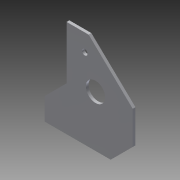
# Autodesk Inventor part: OutlineSketch1
Saved by Autodesk Inventor 2013 (Build 170138000, 138)
## iProperties
Created: 2013-06-03
Part Number: OutlineSketch1
Material: Aluminum 6061
Document SubType Name: Modeling
Designer: mvarma
Density: 1 g/cm^3
Author: mvarma
Autodesk Inventor part; units mm, degrees
ref_plane "YZ Plane" through (0, 0, 0) normal (1, 0, 0) x (0, 1, 0)
ref_plane "XZ Plane" through (0, 0, 0) normal (0, 1, 0) x (-1, 0, 0)
ref_plane "XY Plane" through (0, 0, 0) normal (0, 0, 1) x (1, 0, 0)
sketch "Sketch1" plane through (0, 0, 0) normal (0, 0, 1) x (1, 0, 0)
  line L0 (0, 0) -> (304.8, 0) construction
  line L1 (304.8, 0) -> (304.8, 50.8) construction
  line L2 (304.8, 50.8) -> (0, 50.8) construction
  line L3 (0, 50.8) -> (0, 0) construction
  circle A0 centre (152.4, 25.4) radius 14.2875 construction
  circle A1 centre (152.4, 25.4) radius 30.48 construction
  circle A2 centre (152.4, 25.4) radius 22.225 construction
  line L4 (152.4, 25.4) -> (138.5082, 62.9697) construction
  circle A3 centre (138.5082, 62.9697) radius 9.525 construction
  circle A4 centre (138.5082, 62.9697) radius 17.78 construction
  circle A5 centre (89.9711, 85.09) radius 31.75 construction
  circle A6 centre (160.9785, 111.3458) radius 31.75 construction
  circle A7 centre (221.9701, 85.09) radius 31.75 construction
  line L5 (0, 50.8) -> (0, 53.34) construction
  line L6 (0, 53.34) -> (304.8, 53.34) construction
  line L7 (304.8, 53.34) -> (304.8, 50.8) construction
  circle A8 centre (138.5082, 62.9697) radius 21.59 construction
  circle A9 centre (152.4, 25.4) radius 46.99 construction
  circle A10 centre (152.4, 25.4) radius 50.8 construction
  arc A11 (84.9408, 79.3264) -> (90.9184, 92.6811) centre (89.9711, 85.09) ccw construction
  circle A12 centre (160.9785, 111.3458) radius 7.65 construction
  arc A13 (221.6946, 92.735) -> (225.5172, 78.312) centre (221.9701, 85.09) ccw construction
  circle A14 centre (160.9785, 111.3458) radius 9.1 construction
  circle A15 centre (138.5082, 62.9697) radius 22.9 construction
  line L8 (84.9408, 79.3264) -> (123.4503, 45.7166) construction
  line L9 (168.5483, 110.2412) -> (161.1682, 59.6633) construction
  line L10 (90.9184, 92.6811) -> (89.9711, 85.09) construction
  line L11 (89.9711, 85.09) -> (84.9408, 79.3264) construction
  circle A16 centre (126.192, 96.2783) radius 3.175
  circle A17 centre (126.192, 96.2783) radius 7.9375 construction
  line L12 (90.9184, 92.6811) -> (125.2091, 88.4019) construction
  line L13 (132.0626, 90.936) -> (155.3205, 116.4945) construction
  line L14 (155.3205, 116.4945) -> (160.9785, 111.3458) construction
  line L15 (168.5483, 110.2412) -> (160.9785, 111.3458) construction
  line L16 (138.5082, 62.9697) -> (126.192, 96.2783) construction
  line L17 (89.9711, 85.09) -> (160.9785, 111.3458) construction
  line L18 (152.4, 25.4) -> (89.9711, 85.09) construction
  line L19 (152.4, 25.4) -> (160.9785, 111.3458) construction
  circle A18 centre (126.192, 96.2783) radius 9.2075 construction
  circle A19 centre (126.192, 96.2783) radius 6.1595 construction
  arc A20 (90.9184, 92.6811) -> (84.9408, 79.3264) centre (89.9711, 85.09) ccw construction
  circle A21 centre (160.9785, 111.3458) radius 25.4 construction
  circle A22 centre (221.9701, 85.09) radius 25.4 construction
  line L20 (102.9424, 114.0695) -> (76.9998, 56.1105) construction
  circle A23 centre (89.9711, 85.09) radius 25.4 construction
  line L21 (213.8361, 115.7804) -> (230.1041, 54.3996) construction
  line L22 (54.4111, 146.9058) -> (257.6111, 146.9058)
  line L23 (257.6111, 146.9058) -> (257.6111, -11.8442)
  line L24 (257.6111, -11.8442) -> (54.4111, -11.8442)
  line L25 (54.4111, -11.8442) -> (54.4111, 146.9058)
  circle A24 centre (138.5082, 62.9697) radius 11.1125
  arc A25 (225.3129, 75.4455) -> (221.0936, 95.3227) centre (223.2033, 85.3841) ccw construction
  line L26 (220.7531, 84.7347) -> (228.4773, 60.5377) construction
  line L27 (223.2033, 85.3841) -> (228.4773, 60.5377) construction
  line L28 (220.7531, 84.7347) -> (213.029, 108.9318) construction
  line L29 (223.2033, 85.3841) -> (217.9292, 110.2305) construction
  arc A26 (212.3049, 111.2003) -> (213.7531, 106.6633) centre (213.029, 108.9318) ccw construction
  arc A27 (218.4237, 107.9012) -> (217.4348, 112.5599) centre (217.9292, 110.2305) ccw construction
  arc A28 (218.4237, 107.9012) -> (213.7531, 106.6633) centre (228.4773, 60.5377) ccw construction
  arc A29 (217.4348, 112.5599) -> (212.3049, 111.2003) centre (228.4773, 60.5377) ccw construction
  line L30 (213.029, 108.9318) -> (212.3049, 111.2003) construction
  line L31 (217.9292, 110.2305) -> (217.4348, 112.5599) construction
  arc A30 (221.0936, 95.3227) -> (217.6635, 94.4136) centre (228.4773, 60.5377) ccw construction
  arc A31 (225.3129, 75.4455) -> (223.8428, 75.0559) centre (228.4773, 60.5377) ccw construction
  line L32 (102.6358, 107.1803) -> (91.1149, 84.5434) construction
  line L33 (79.5941, 61.9064) -> (88.8014, 85.5789) construction
  arc A32 (98.8719, 111.4706) -> (97.1455, 107.0321) centre (98.0087, 109.2513) ccw construction
  arc A33 (101.5557, 105.0581) -> (103.7158, 109.3025) centre (102.6358, 107.1803) ccw construction
  arc A34 (101.5557, 105.0581) -> (97.1455, 107.0321) centre (79.5941, 61.9064) ccw construction
  line L34 (98.0087, 109.2513) -> (98.8719, 111.4706) construction
  line L35 (102.6358, 107.1803) -> (103.7158, 109.3025) construction
  arc A35 (103.7158, 109.3025) -> (98.8719, 111.4706) centre (79.5941, 61.9064) ccw construction
  arc A36 (217.6635, 94.4136) -> (223.8428, 75.0559) centre (220.7531, 84.7347) ccw construction
  arc A37 (86.5066, 75.4886) -> (95.7233, 93.5981) centre (91.1149, 84.5434) ccw construction
  line L36 (88.8014, 85.5789) -> (98.0087, 109.2513) construction
  line L37 (91.1149, 84.5434) -> (79.5941, 61.9064) construction
  arc A38 (86.5066, 75.4886) -> (85.1185, 76.1099) centre (79.5941, 61.9064) ccw construction
  arc A39 (95.7233, 93.5981) -> (92.4843, 95.0479) centre (79.5941, 61.9064) ccw construction
  arc A40 (92.4843, 95.0479) -> (85.1185, 76.1099) centre (88.8014, 85.5789) ccw construction
  line L38 (160.9785, 111.3458) -> (138.0151, 122.2014) construction
  line L39 (160.9785, 111.3458) -> (183.9418, 100.4902) construction
  circle A41 centre (138.5082, 62.9697) radius 26.75 construction
  line L40 (221.6946, 92.735) -> (137.5448, 89.7024) construction
  line L41 (225.5172, 78.312) -> (150.9113, 39.269) construction
  line L42 (221.9701, 85.09) -> (221.6946, 92.735) construction
  line L43 (221.9701, 85.09) -> (225.5172, 78.312) construction
  line L44 (138.5082, 62.9697) -> (137.5448, 89.7024) construction
  line L45 (138.5082, 62.9697) -> (150.9113, 39.269) construction
  arc A42 (225.5172, 78.312) -> (221.6946, 92.735) centre (221.9701, 85.09) ccw construction
  arc A43 (225.5172, 78.312) -> (224.7763, 77.9733) centre (221.9701, 85.09) ccw construction
  line L46 (138.5082, 62.9697) -> (221.9701, 85.09) construction
  line L47 (79.8111, 29.4308) -> (105.2111, 54.8308)
  line L48 (105.2111, 54.8308) -> (105.2111, 116.102)
  line L49 (105.2111, 116.102) -> (130.6111, 116.102)
  line L50 (130.6111, 116.102) -> (181.4111, 67.5308)
  line L51 (181.4111, 67.5308) -> (181.4111, 29.4308)
  line L52 (156.0111, 4.0308) -> (79.8111, 4.0308)
  line L53 (79.8111, 4.0308) -> (79.8111, 29.4308)
  line L54 (156.0111, 4.0308) -> (181.4111, 29.4308)
  point P0 (215.4629, 109.6423)
  point P1 (100.3481, 108.2736)
  dimension "d1" = 50.8
  dimension "d2" = 28.575
  dimension "d3" = 25.4
  dimension "d4" = 152.4
  dimension "d7" = 60.96
  dimension "d8" = 44.45
  dimension "d9" = 19.05
  dimension "d10" = 35.56
  dimension "d11" = 40.0558
  dimension "d12" = 63.5
  dimension "d13" = 63.5
  dimension "d14" = 63.5
  dimension "d15" = 2.54
  dimension "d16" = 304.8
  dimension "d17" = 43.18
  dimension "d18" = 93.98
  dimension "d19" = 101.6
  dimension "d21" = 15.3
  dimension "d22" = 15.3
  dimension "d24" = 18.2
  dimension "d29" = 45.8
  dimension "d30" = 146
  dimension "d31" = 6.35
  dimension "d32" = 15.875
  dimension "d33" = 146
  dimension "d35" = 18.415
  dimension "d37" = 12.319
  dimension "d40" = 50.8
  dimension "d41" = 50.8
  dimension "d42" = 17
  dimension "d43" = 17
  dimension "d44" = 50.8
  dimension "d53" = 203.2
  dimension "d54" = 158.75
  dimension "d55" = 35.56
  dimension "d56" = 35.56
  dimension "d57" = 22.225
  dimension "d67" = 25.4
  dimension "d68" = 25.4
  dimension "d69" = 2.86
  dimension "d70" = 25.4
  dimension "d71" = 25.4
  dimension "d72" = 4.7625
  dimension "d75" = 2.86
  dimension "d80" = 4.7625
  dimension "d82" = 4.7625
  dimension "d83" = 50.8
  dimension "d84" = 50.8
  dimension "d85" = 10.16
  dimension "d97" = 48.4188
  dimension "d99" = 20.32
  dimension "d101" = 25.4
  dimension "d102" = 25.4
  dimension "d103" = 10.16
  dimension "d105" = 17
  dimension "d106" = 17
  dimension "d107" = 53.5
  dimension "d108" = 154.44
  dimension "d109" = 7.65
  dimension "d111" = 86.3435
  dimension "d112" = 12.78
  dimension "d113" = 12.78
  dimension "d116" = 25.4
  dimension "d117" = 25.4
  constraints: 112 end point, 62 point on circle, 44 centre point, 32 coincident, 18 tangent, 14 point on line, 12 perpendicular, 11 parallel, 10 collinear, 2 horizontal, 2 midpoint, 1 equal radius, 3 other
  measures "d1" distance of L1.end L0.end
  measures "d2" diameter of A0
  measures "d3" distance from line of L0 A0.centre
  measures "d4" distance from line of L3 A0.centre
  measures "d7" diameter of A1
  measures "d8" diameter of A2
  measures "d9" diameter of A3
  measures "d10" diameter of A4
  measures "d11" distance of L4.start L4.end
  measures "d12" diameter of A5
  measures "d13" diameter of A6
  measures "d14" diameter of A7
  measures "d15" distance of L2.end L5.end
  measures "d16" distance of L0.end L0.start
  measures "d17" diameter of A8
  measures "d18" diameter of A9
  measures "d19" diameter of A10
  measures "d21" diameter of A11
  measures "d22" diameter of A12
  measures "d24" diameter of A14
  measures "d29" diameter of A15
  measures "d30" angle of L11 L10
  measures "d31" diameter of A16
  measures "d32" diameter of A17
  measures "d33" angle of L15 L14
  measures "d35" diameter of A18
  measures "d37" diameter of A19
  measures "d40" diameter of A21
  measures "d41" diameter of A22
  measures "d42" angle of L10 L20
  measures "d43" angle of L11 L20
  measures "d44" diameter of A23
  measures "d53" distance of L23.end L24.end
  measures "d54" distance of L22.end L23.end
  measures "d55" distance from line of L25 A5.centre
  measures "d56" distance from line of L22 A6.centre
  measures "d57" diameter of A24
  measures "d67" distance of L26.start L26.end
  measures "d68" distance of L27.start L26.end
  measures "d69" angle of L21 L26
  measures "d70" distance of L26.start L28.end
  measures "d71" distance of L27.start L29.end
  measures "d72" diameter of A26
  measures "d75" angle of L20 L32
  measures "d80" diameter of A32
  measures "d82" diameter of A33
  measures "d83" distance of L33.start L36.end
  measures "d84" distance of L32.start L33.start
  measures "d85" radius of A25
  measures "d97" radius of A34
  measures "d99" diameter of A37
  measures "d101" distance of L33.start L33.end
  measures "d102" distance of L32.end L33.start
  measures "d103" radius of A40
  measures "d105" angle of L38 L14
  measures "d106" angle of L39 L15
  measures "d107" diameter of A41
  measures "d108" angle of L42 L43
  measures "d109" radius of A13
  measures "d111" distance of L44.start L42.start
  measures "d112" angle of L21 L42
  measures "d113" angle of L21 L43
  measures "d116" distance of L48.end L49.end
  measures "d117" horizontal distance of L47.start L47.end
extrude "Extrusion3" add sketch "Sketch1" along normal blind 3.175 contours L47 L48 L49 L50 L51 L54 L52 L53
equation "\"d2\" = BearingLargeOD"
equation "\"d7\" = Gear48tPD"
equation "\"d8\" = Gear35tPD"
equation "\"d9\" = Gear15tPD"
equation "\"d10\" = Gear28tPD"
equation "\"d11\" = 0.5 * Gear48tPD + 0.5 * Gear15tPD + MeshingClearance"
equation "\"d12\" = CimOD"
equation "\"d13\" = CimOD"
equation "\"d14\" = CimOD"
equation "\"d17\" = Gear28tPD + ClearanceDiameter"
equation "\"d18\" = WheelOD"
equation "\"d19\" = WheelClearance"
equation "\"Pulley48tPD\" = 45.8"
equation "\"Pulley19tPD\" = 18.2"
equation "\"Pulley16tPD\" = 15.3"
equation "\"Gear15tPD\" = 19.05"
equation "\"Gear35tPD\" = 44.45"
equation "\"Gear48tPD\" = 60.96"
equation "\"Gear28tPD\" = 35.56"
equation "\"BearingLargeOD\" = 28.575"
equation "\"BearingSmallOD\" = 22.225"
equation "\"MeshingClearance\" = 0.0508"
equation "\"CimOD\" = 63.5"
equation "\"WheelOD\" = 93.98"
equation "\"ClearanceDiameter\" = 7.62"
equation "\"WheelClearance\" = 101.6"
equation "\"TensioningBearingID\" = 6.35"
equation "\"TensioningBearingOD\" = 15.875"
equation "\"SpingClipClearance\" = 8.89"
equation "\"Pi\" = 79.79645"
equation "\"Pulley56tPD\" = 53.5"
equation "\"BearingXLargeOD\" = 34.925"
body "Solid3"
